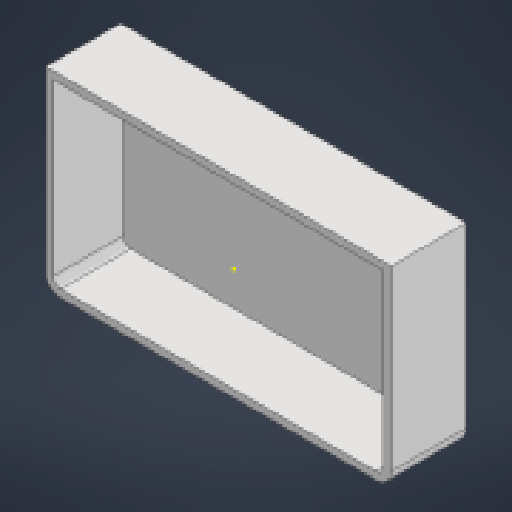
# Autodesk Inventor part: 后盖电路
Saved by Autodesk Inventor 2025 (Build 290162000, 162)
## iProperties
Created: 2025-12-26
Part Number: 后盖电路
Material: 常规
Document SubType Name: Modeling
Designer: XH
Density: 1 g/cm^3
Appearance: 默认
Author: XH
Autodesk Inventor part; units mm, degrees
ref_plane "YZ Plane" through (0, 0, 0) normal (1, 0, 0) x (0, 1, 0)
ref_plane "XZ Plane" through (0, 0, 0) normal (0, 1, 0) x (-1, 0, 0)
ref_plane "XY Plane" through (0, 0, 0) normal (0, 0, 1) x (1, 0, 0)
sketch "草图1" plane through (0, 0, 0) normal (0, 0, 1) x (1, 0, 0)
  line L0 (-69.1834, -44.3704) -> (56.8166, -44.3704)
  arc A0 (56.8166, -44.3704) -> (62.8166, -38.3704) centre (56.8166, -38.3704) ccw
  line L1 (62.8166, 27.5796) -> (62.8166, -38.3704)
  line L2 (62.8166, 27.5796) -> (62.8166, 32.6296)
  line L3 (62.8166, 32.6296) -> (-75.1834, 32.6296)
  line L4 (-75.1834, -38.3704) -> (-75.1834, 32.6296)
  arc A1 (-75.1834, -38.3704) -> (-69.1834, -44.3704) centre (-69.1834, -38.3704) ccw
  constraints: 10 end point, 4 point on circle, 2 centre point, 2 other
extrude "拉伸1" add sketch "草图1" along normal blind 30
sketch "草图2" plane through (0, 0, 30) normal (0, 0, 1) x (1, 0, 0)
  point P0 (0, 0)
sketch "草图3" plane through (0, 0, 30) normal (0, 0, 1) x (1, 0, 0)
  line L0 (-69.1834, -44.3704) -> (56.8166, -44.3704) projected
  arc A0 (-75.1834, -38.3704) -> (-69.1834, -44.3704) centre (-69.1834, -38.3704) ccw projected
  line L1 (-75.1834, 32.6296) -> (-75.1834, -38.3704) projected
  line L2 (62.8166, 32.6296) -> (-75.1834, 32.6296) projected
  line L3 (62.8166, -38.3704) -> (62.8166, 32.6296) projected
  arc A1 (56.8166, -44.3704) -> (62.8166, -38.3704) centre (56.8166, -38.3704) ccw projected
  line L4 (-69.1834, -41.3704) -> (56.8166, -41.3704)
  arc A2 (56.8166, -41.3704) -> (59.8166, -38.3704) centre (56.8166, -38.3704) ccw
  line L5 (59.8166, -38.3704) -> (59.8166, 29.6296)
  line L6 (59.8166, 29.6296) -> (-72.1834, 29.6296)
  line L7 (-72.1834, 29.6296) -> (-72.1834, -38.3704)
  arc A3 (-72.1834, -38.3704) -> (-69.1834, -41.3704) centre (-69.1834, -38.3704) ccw
  point P0 (0, 0)
  dimension "d3" = 3
  constraints: 8 end point, 4 point on circle, 2 centre point, 5 other
  measures "d3" radial gap between concentric circles of A0 A3
extrude "拉伸2" cut sketch "草图3" against normal blind 28 contours A3 L7 L6 L5 A2 L4
